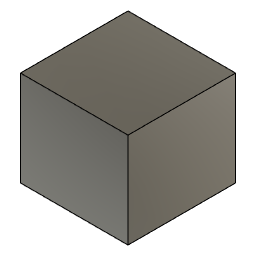
tp_cap v1 (Autodesk Fusion 360 design; units mm, degrees)
Autodesk Fusion 360 part; units mm, degrees
sketch "Sketch1" plane through (0, 0, 0) normal (0, 0, 1) x (1, 0, 0)
  line L0 (0, 0) -> (4.52, 0)
  line L1 (4.52, 0) -> (4.52, 4.52)
  line L2 (4.52, 4.52) -> (0, 4.52)
  line L3 (0, 4.52) -> (0, 0)
  line L4 (0, 4.52) -> (4.52, 0) construction
  line L5 (4.52, 4.52) -> (0, 0) construction
  circle A0 centre (2.26, 2.26) radius 1.2
  dimension "d1" = 4.52
  dimension "d2" = 4.52
  dimension "d3" = 2.4
  constraint horizontal L0
  constraint vertical L1
  constraint horizontal L2
  constraint vertical L3
  constraint coincident L0.start L3.end
  constraint midpoint L5 A0.centre
  measures "d1" distance of L0.start L0.end
  measures "d2" distance of L0.start L2.end
  measures "d3" diameter of A0
extrude "Extrude1" add sketch "Sketch1" along normal blind 3
sketch "Sketch2" plane through (0, 0, 3) normal (0, 0, 1) x (-1, 0, 0)
  circle A0 centre (-2.26, -2.26) radius 1.2
  line L0 (0, -4.52) -> (0, 0)
  line L1 (0, 0) -> (-4.52, 0)
  line L2 (-4.52, 0) -> (-4.52, -4.52)
  line L3 (-4.52, -4.52) -> (0, -4.52)
extrude "Extrude2" add sketch "Sketch2" along normal blind 1 contours A0 | L0 L1 L2 L3
